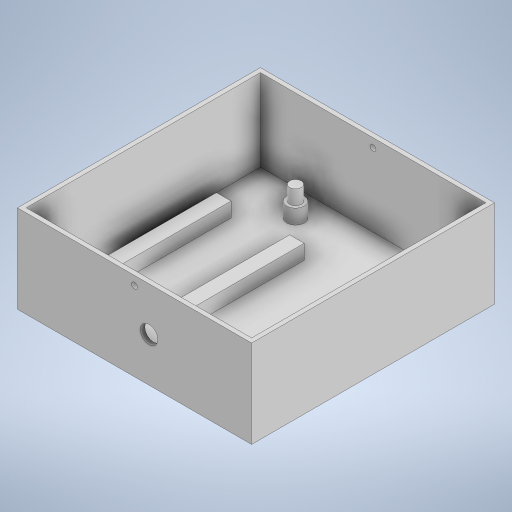
# Autodesk Inventor part: Gyrosensor
Saved by Autodesk Inventor 2024 (Build 280153000, 153)
## iProperties
Created: 2024-01-17
Part Number: Gyrosensor
Material: Generisch
Document SubType Name: Modeling
Designer: User
Density: 1 g/cm^3
Appearance: Vorgabe
Author: User
Autodesk Inventor part; units mm, degrees
ref_plane "YZ Plane" through (0, 0, 0) normal (1, 0, 0) x (0, 1, 0)
ref_plane "XZ Plane" through (0, 0, 0) normal (0, 1, 0) x (-1, 0, 0)
ref_plane "XY Plane" through (0, 0, 0) normal (0, 0, 1) x (1, 0, 0)
sketch "Skizze1" plane through (0, 0, 0) normal (0, 0, 1) x (1, 0, 0)
  line L0 (0, 0) -> (80, 0)
  line L1 (80, 0) -> (80, 83)
  line L2 (80, 83) -> (0, 83)
  line L3 (0, 83) -> (0, 0)
  line L4 (1.5, 81.5) -> (78.5, 81.5)
  line L5 (78.5, 81.5) -> (78.5, 1.5)
  line L6 (78.5, 1.5) -> (1.5, 1.5)
  line L7 (1.5, 1.5) -> (1.5, 81.5)
  dimension "d0" = 80
  dimension "d1" = 83
  dimension "d2" = 1.5
  dimension "d3" = 1.5
  dimension "d4" = 1.5
  dimension "d5" = 1.5
  constraints: 16 end point, 4 parallel, 2 horizontal, 2 perpendicular
  measures "d0" distance of L2.end L1.end
  measures "d1" distance of L1.end L0.end
  measures "d2" distance between parallel lines of L2 L4
  measures "d3" distance between parallel lines of L3 L7
  measures "d4" distance between parallel lines of L0 L6
  measures "d5" distance between parallel lines of L1 L5
extrude "Extrusion1" add sketch "Skizze1" along normal blind 2 contours L4 L5 L6 L7
extrude "Extrusion2" add sketch "Skizze1" along normal blind 30
sketch "Skizze2" plane through (0, 0, 2) normal (0, 0, 1) x (1, 0, 0)
  circle A0 centre (22.5, 72.5) radius 3
  circle A1 centre (21, 10.5) radius 3
  line L0 (1.5, 1.5) -> (1.5, 81.5) projected
  circle A2 centre (22.5, 72.5) radius 2
  circle A3 centre (21, 10.5) radius 2
  circle A4 centre (65.5, 41.5) radius 1
  circle A5 centre (65.5, 41.5) radius 2.5
  line L1 (78.5, 81.5) -> (78.5, 1.5) projected
  line L2 (78.5, 1.5) -> (1.5, 1.5) projected
  line L3 (1.5, 81.5) -> (78.5, 81.5) projected
  line L4 (31.5, 21.5) -> (36.5, 21.5)
  line L5 (36.5, 21.5) -> (36.5, 61.5)
  line L6 (36.5, 61.5) -> (31.5, 61.5)
  line L7 (31.5, 61.5) -> (31.5, 21.5)
  line L8 (6.5, 21.5) -> (11.5, 21.5)
  line L9 (11.5, 21.5) -> (11.5, 61.5)
  line L10 (11.5, 61.5) -> (6.5, 61.5)
  line L11 (6.5, 61.5) -> (6.5, 21.5)
  line L12 (61, 10.5) -> (71, 10.5)
  line L13 (71, 10.5) -> (71, 20.5)
  line L14 (71, 20.5) -> (61, 20.5)
  line L15 (61, 20.5) -> (61, 10.5)
  line L16 (61, 60.5117) -> (71, 60.5117)
  line L17 (71, 60.5117) -> (71, 70.5117)
  line L18 (71, 70.5117) -> (61, 70.5117)
  line L19 (61, 70.5117) -> (61, 60.5117)
  point P0 (0, 0)
  point P1 (71, 65.5117)
  dimension "d11" = 21
  dimension "d12" = 19.5
  dimension "d13" = 4
  dimension "d14" = 4
  dimension "d15" = 6
  dimension "d16" = 6
  dimension "d17" = 2
  dimension "d18" = 5
  dimension "d23" = 13
  dimension "d31" = 62
  dimension "d32" = 9
  dimension "d33" = 9
  dimension "d44" = 5
  dimension "d45" = 40
  dimension "d46" = 30
  dimension "d47" = 20
  dimension "d48" = 20
  dimension "d49" = 5
  dimension "d50" = 40
  dimension "d51" = 20
  dimension "d52" = 5
  dimension "d53" = 10
  dimension "d54" = 10
  dimension "d55" = 10
  dimension "d56" = 10
  dimension "d57" = 7.5
  dimension "d58" = 7.5
  constraints: 32 end point, 8 parallel, 6 centre point, 4 horizontal, 4 perpendicular, 3 coincident, 1 midpoint
  measures "d11" distance from line of L0 A0.centre
  measures "d12" distance from line of L0 A1.centre
  measures "d13" diameter of A2
  measures "d14" diameter of A3
  measures "d15" diameter of A0
  measures "d16" diameter of A1
  measures "d17" diameter of A4
  measures "d18" diameter of A5
  measures "d23" distance from line of A4.centre L1
  measures "d31" vertical distance of A1.centre A0.centre
  measures "d32" distance from line of L2 A1.centre
  measures "d33" distance from line of L3 A0.centre
  measures "d44" distance of L6.end L5.end
  measures "d45" distance of L5.end L4.end
  measures "d46" distance between parallel lines of L0 L7
  measures "d47" distance between parallel lines of L3 L6
  measures "d48" distance between parallel lines of L2 L4
  measures "d49" distance of L10.end L10.start
  measures "d50" distance of L10.start L8.end
  measures "d51" distance between parallel lines of L3 L10
  measures "d52" distance between parallel lines of L0 L11
  measures "d53" distance of L14.end L13.end
  measures "d54" distance of L13.end L12.end
  measures "d55" distance of L18.end L17.end
  measures "d56" distance of L17.end L16.end
  measures "d57" distance from line of L1 point (71, 65.512)
  measures "d58" distance between parallel lines of L1 L13
extrude "Extrusion3" add sketch "Skizze2" along normal blind 5 contours A0 | A1 | A5 | L7 L6 L5 L4 | L11 L10 L9 L8 | L15 L14 L13 L12 | L19 L18 L17 L16
extrude "Extrusion4" add sketch "Skizze2" along normal blind 10 contours A2 | A3
sketch "Skizze4" plane through (0, 0, 0) normal (0, -1, 0) x (1, 0, 0)
  circle A0 centre (40, 27) radius 1
  line L0 (0, 30) -> (80, 30) projected
  line L1 (0, 0) -> (0, 30) projected
  dimension "d34" = 2
  dimension "d35" = 3
  dimension "d36" = 40
  constraints: 1 centre point
  measures "d34" diameter of A0
  measures "d35" distance from line of L0 A0.centre
  measures "d36" distance from line of L1 A0.centre
extrude "Extrusion6" cut sketch "Skizze4" against normal through all
sketch "Skizze5" plane through (0, 0, 0) normal (0, -1, 0) x (1, 0, 0)
  circle A0 centre (45, 15) radius 3
  line L0 (0, 0) -> (0, 30) projected
  line L1 (0, 30) -> (80, 30) projected
  dimension "d39" = 6
  dimension "d40" = 45
  dimension "d41" = 15
  constraints: 1 centre point
  measures "d39" diameter of A0
  measures "d40" distance from line of L0 A0.centre
  measures "d41" distance from line of L1 A0.centre
extrude "Extrusion7" cut sketch "Skizze5" against normal blind 5
